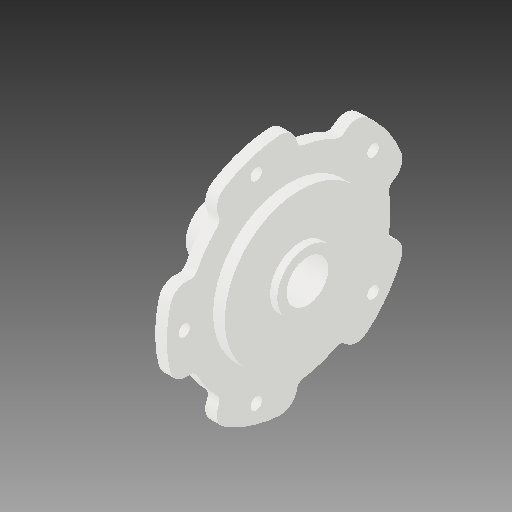
# Autodesk Inventor part: 362-03
Saved by Autodesk Inventor 2019 (Build 230136000, 136)
## iProperties
Company: Autodesk Inc.
Created: 2017-03-19
Part Number: 362-03
Material: Generic
Document SubType Name: Modeling
Designer: Autodesk Inc.
Density: 1 g/cm^3
Appearance: Default
Mass: 60.6838 g
Surface Area: 218.504 cm^2
Volume: 60.6838 cm^3
Author: Inventor
Autodesk Inventor part; units mm, degrees
ref_plane "YZ Plane" through (0, 0, 0) normal (1, 0, 0) x (0, 1, 0)
ref_plane "XZ Plane" through (0, 0, 0) normal (0, 1, 0) x (-1, 0, 0)
ref_plane "XY Plane" through (0, 0, 0) normal (0, 0, 1) x (1, 0, 0)
sketch "Sketch2" plane through (0, 0, 0) normal (1, 0, 0) x (0, 1, 0)
  arc A0 (12.5, 50.9902) -> (-12.5, 50.9902) centre (0, 0) ccw
  arc A1 (-19.5, 39.443) -> (-17.7114, 42.7254) centre (-20.9403, 42.3564) ccw
  line L0 (-17.7114, 42.7254) -> (-17.7881, 43.3968)
  arc A2 (-12.5, 50.9902) -> (-17.7881, 43.3968) centre (-10.8333, 44.1915) ccw
  line L1 (0, 0) -> (0, 52.5) construction
  arc A3 (17.7114, 42.7254) -> (19.5, 39.443) centre (20.9403, 42.3564) ccw
  line L2 (17.7114, 42.7254) -> (17.7881, 43.3968)
  arc A4 (17.7881, 43.3968) -> (12.5, 50.9902) centre (10.8333, 44.1915) ccw
  arc A5 (-44.6318, 27.645) -> (-52.3573, 3.8686) centre (0, 0) ccw
  arc A6 (-43.5384, -6.357) -> (-46.1074, -3.6416) centre (-46.7543, -6.8266) ccw
  line L3 (-46.1074, -3.6416) -> (-46.7696, -3.5071)
  arc A7 (-52.3573, 3.8686) -> (-46.7696, -3.5071) centre (-45.3763, 3.3528) ccw
  line L4 (0, 0) -> (-49.9305, 16.2234) construction
  arc A8 (-35.776, 30.3278) -> (-44.6318, 27.645) centre (-38.6809, 23.959) ccw
  line L5 (-35.1611, 30.0474) -> (-35.776, 30.3278)
  arc A9 (-35.1611, 30.0474) -> (-31.4867, 30.7342) centre (-33.8124, 33.0043) ccw
  arc A10 (-40.084, -33.9046) -> (-19.8586, -48.5993) centre (0, 0) ccw
  arc A11 (-7.4082, -43.3719) -> (-10.7846, -44.976) centre (-7.9554, -46.5755) ccw
  line L6 (-10.7846, -44.976) -> (-11.1171, -45.5643)
  arc A12 (-19.8586, -48.5993) -> (-11.1171, -45.5643) centre (-17.2108, -42.1194) ccw
  line L7 (0, 0) -> (-30.8587, -42.4734) construction
  arc A13 (-39.8989, -24.6532) -> (-40.084, -33.9046) centre (-34.7395, -29.384) ccw
  line L8 (-39.4421, -24.1551) -> (-39.8989, -24.6532)
  arc A14 (-39.4421, -24.1551) -> (-38.9598, -20.4482) centre (-41.8376, -21.9586) ccw
  arc A15 (19.8586, -48.5993) -> (40.084, -33.9046) centre (0, 0) ccw
  arc A16 (38.9598, -20.4482) -> (39.4421, -24.1551) centre (41.8376, -21.9586) ccw
  line L9 (39.4421, -24.1551) -> (39.8989, -24.6532)
  arc A17 (40.084, -33.9046) -> (39.8989, -24.6532) centre (34.7395, -29.384) ccw
  line L10 (0, 0) -> (30.8587, -42.4734) construction
  arc A18 (11.1171, -45.5643) -> (19.8586, -48.5993) centre (17.2108, -42.1194) ccw
  line L11 (10.7846, -44.976) -> (11.1171, -45.5643)
  arc A19 (10.7846, -44.976) -> (7.4082, -43.3719) centre (7.9554, -46.5755) ccw
  arc A20 (52.3573, 3.8686) -> (44.6318, 27.645) centre (0, 0) ccw
  arc A21 (31.4867, 30.7342) -> (35.1611, 30.0474) centre (33.8124, 33.0043) ccw
  line L12 (35.1611, 30.0474) -> (35.776, 30.3278)
  arc A22 (44.6318, 27.645) -> (35.776, 30.3278) centre (38.6809, 23.959) ccw
  line L13 (0, 0) -> (49.9305, 16.2234) construction
  arc A23 (46.7696, -3.5071) -> (52.3573, 3.8686) centre (45.3763, 3.3528) ccw
  line L14 (46.1074, -3.6416) -> (46.7696, -3.5071)
  arc A24 (46.1074, -3.6416) -> (43.5384, -6.357) centre (46.7543, -6.8266) ccw
  arc A25 (38.9598, -20.4482) -> (43.5384, -6.357) centre (0, 0) ccw
  arc A26 (-7.4082, -43.3719) -> (7.4082, -43.3719) centre (0, 0) ccw
  arc A27 (-43.5384, -6.357) -> (-38.9598, -20.4482) centre (0, 0) ccw
  arc A28 (31.4867, 30.7342) -> (19.5, 39.443) centre (0, 0) ccw
  arc A29 (-19.5, 39.443) -> (-31.4867, 30.7342) centre (0, 0) ccw
  dimension "d75" = 52.5
  dimension "d76" = 7
  dimension "d77" = 3.25
  dimension "d80" = 360
  dimension "d83" = 44
  dimension "d84" = 12.5
  dimension "d85" = 19.5
  constraints: 77 point on circle, 30 centre point, 30 end point, 6 symmetric about line, 5 coincident, 5 tangent, 1 vertical, 142 other
  measures "d75" radius of A0
  measures "d76" radius of A2
  measures "d77" radius of A1
  measures "d83" radius of A28
  measures "d84" distance from line of L1 A0.end
  measures "d85" distance from line of L1 A1.start
extrude "Extrusion1" add sketch "Sketch2" along normal blind 5
sketch "Sketch3" plane through (0, 0, 0) normal (-1, 0, 0) x (0, 0, 1)
  circle A0 centre (0, 0) radius 11.5
  circle A1 centre (0, 0) radius 9
  point P0 (0, 0)
  dimension "d55" = 23
  dimension "d56" = 18
  constraints: 2 centre point, 1 coincident, 1 concentric
  measures "d55" diameter of A0
  measures "d56" diameter of A1
extrude "Extrusion2" add sketch "Sketch3" along normal blind 27.81
fillet "Fillet1" radius 14 1 edges at (0, 0, -11.5)
sketch "Sketch4" plane through (5, 0, 0) normal (1, 0, 0) x (0, 0, -1)
  circle A0 centre (0, 0) radius 32.5
  point P0 (0, 0)
  dimension "d60" = 65
  constraints: 1 centre point, 1 coincident
  measures "d60" diameter of A0
extrude "Extrusion3" add sketch "Sketch4" along normal blind 5
sketch "Sketch5" plane through (10, 0, 0) normal (1, 0, 0) x (0, 0, -1)
  circle A0 centre (0, 0) radius 13
  point P0 (0, 0)
  dimension "d63" = 26
  constraints: 1 centre point, 1 coincident
  measures "d63" diameter of A0
extrude "Extrusion4" add sketch "Sketch5" along normal blind 3.108
sketch "Sketch6" plane through (13.108, 0, 0) normal (1, 0, 0) x (0, 0, -1)
  circle A0 centre (0, 0) radius 9 projected
  point P0 (0, 0)
extrude "Extrusion5" cut sketch "Sketch6" against normal through all
sketch "Sketch7" plane through (5, 0, 0) normal (1, 0, 0) x (0, 0, -1)
  circle A0 centre (-45, 0) radius 2.5
  point P0 (0, 0)
  dimension "d68" = 45
  dimension "d69" = 5
  constraints: 1 centre point
  measures "d68" distance of point (0, 0) A0.centre
  measures "d69" diameter of A0
extrude "Extrusion6" cut sketch "Sketch7" against normal through all
pattern_circular "Circular Pattern1" count 5 over 360 about axis through (-10, 0, 0) along (1, 0, 0) of "Extrusion6"
body "Solid1"
